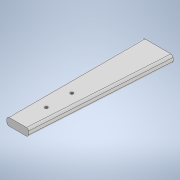
# Autodesk Inventor part: Brillenbuegel
Saved by Autodesk Inventor 2020 (Build 240168000, 168)
## iProperties
Created: 2020-03-19
Part Number: Brillenbuegel
Material: Generisch
Document SubType Name: Modeling
Designer: Fynn
Density: 1 g/cm^3
Appearance: Vorgabe
Author: Fynn
Autodesk Inventor part; units mm, degrees
ref_plane "YZ Plane" through (0, 0, 0) normal (1, 0, 0) x (0, 1, 0)
ref_plane "XZ Plane" through (0, 0, 0) normal (0, 1, 0) x (-1, 0, 0)
ref_plane "XY Plane" through (0, 0, 0) normal (0, 0, 1) x (1, 0, 0)
sketch "Skizze1" plane through (0, 0, 0) normal (0, 1, 0) x (-1, 0, 0)
  line L0 (0, 0) -> (10.3, 0)
  line L1 (10.3, 0) -> (10.3, -65)
  line L2 (10.3, -65) -> (-4.1, -65)
  line L3 (-4.1, -65) -> (0, 0)
  dimension "d0" = 65
  dimension "d1" = 14.4
  dimension "d2" = 10.3
  constraints: 8 end point, 2 perpendicular, 1 horizontal
  measures "d0" distance of L0.end L1.end
  measures "d1" distance of L1.end L2.end
  measures "d2" distance of L0.start L0.end
extrude "Extrusion1" add sketch "Skizze1" along normal blind 3.6
sketch "Skizze2" plane through (0, 3.6, 0) normal (0, 1, 0) x (1, 0, 0)
  line L0 (-10.3, 65) -> (-10.3, 0) projected
  line L1 (-10.3, 0) -> (-10.3, 13)
  line L2 (-10.3, 0) -> (-10.3, 25)
  line L3 (-10.3, 13) -> (-4.5, 13)
  line L4 (-10.3, 25) -> (-4.3, 25)
  point P0 (0, 0)
  dimension "d5" = 13
  dimension "d6" = 25
  dimension "d7" = 5.8
  dimension "d8" = 6
  constraints: 8 end point, 2 point on line, 1 horizontal, 1 perpendicular
  measures "d5" distance of L0.end L1.end
  measures "d6" distance of L0.end L2.end
  measures "d7" distance of L1.end L3.end
  measures "d8" distance of L2.end L4.end
hole "Bohrung1" at (-4.5, 3.6, -13) at (-4.3, 3.6, -25) direction (0, -1, 0) diameter 1.4 end through all
fillet "Rundung1" radius 1 4 edges at (-10.3, 3.6, -32.5) (-10.3, 0, -32.5) (2.05, 3.6, -32.5) (2.05, 0, -32.5)
